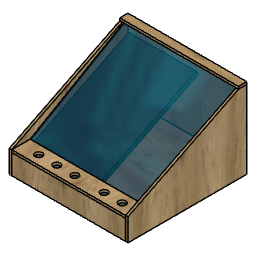
Zeitmaschine (Autodesk Fusion 360 design; units mm, degrees)
Autodesk Fusion 360 part; units mm, degrees
sketch "Skizze1" plane through (0, 0, 0) normal (0, 1, 0) x (1, 0, 0)
  line L0 (0, 0) -> (580, 0)
  line L1 (580, 0) -> (580, 580)
  line L2 (580, 580) -> (0, 580)
  line L3 (0, 580) -> (0, 0)
  line L4 (12, 12) -> (568, 12)
  line L5 (568, 12) -> (568, 568)
  line L6 (568, 568) -> (12, 568)
  line L7 (12, 568) -> (12, 12)
  line L8 (290, 0) -> (290, 580) construction
  dimension "d1" = 580
  dimension "d2" = -12
  constraint horizontal L0
  constraint vertical L1
  constraint horizontal L2
  constraint vertical L3
  constraint coincident L0.start L3.end
  constraint equal L1 L2
  constraint midpoint L0 L8.start
  constraint midpoint L2 L8.end
  measures "d1" distance of L0.end L1.end
sketch "Skizze2" plane through (0, 0, 0) normal (1, 0, 0) x (0, 0, -1)
  line L0 (0, 0) -> (0, 80)
  line L1 (0, 80) -> (100, 80)
  line L2 (100, 80) -> (540, 350)
  line L3 (540, 350) -> (580, 350)
  line L4 (580, 350) -> (580, 0)
  line L5 (580, 0) -> (0, 0)
  line L6 (580, 444.0725) -> (580, 350)
  line L7 (0, 80) -> (540, 350)
  line L8 (0, 80) -> (580, 435.9091)
  line L9 (580, 435.9091) -> (580, 350)
  point P0 (580, 0)
  dimension "d3" = 100
  dimension "d5" = 40
  dimension "d6" = 80
  dimension "d7" = 350
  constraint coincident L0.start L5.end
  constraint vertical L0
  constraint perpendicular L0 L1
  constraint parallel L1 L3
  constraint vertical L4
  constraint coincident P0 L4.end
  constraint perpendicular L3 L6
  constraint parallel L2 L8
  constraint parallel L4 L9
  measures "d3" distance of L0.end L1.end
  measures "d5" distance of L2.end L3.end
  measures "d6" distance of L0.start L0.end
  measures "d7" distance of L3.end P0
extrude "Extrusion1" add sketch "Skizze2" along normal blind 12 contours L0 L1 L2 L3 L4 L5 | L1 L2 L7 makes body 1
ref_plane "Arbeitsebene1" through (290, 0, -290) normal (1, 0, 0) x (0, 0, -1)
mirror "Spiegeln1" about plane through (290, 0, -290) normal (1, 0, 0) of bodies 1 makes body 2
sketch "Skizze3" plane through (0, 0, -580) normal (0, 0, -1) x (-1, 0, 0)
  line L0 (0, 0) -> (0, 350)
  line L1 (0, 350) -> (-12, 350)
  line L2 (-12, 350) -> (-12, 0)
  line L3 (-12, 0) -> (0, 0)
  line L4 (0, 0) -> (-580, 0)
  line L5 (-580, 0) -> (-580, 350)
  line L6 (-580, 350) -> (0, 350)
  line L7 (0, 350) -> (0, 0)
  line L8 (-12, 0) -> (-12, 350)
  line L9 (-568, 0) -> (-568, 350)
  point P0 (-580, 350)
  constraint horizontal L4
  constraint vertical L5
  constraint horizontal L6
  constraint vertical L7
  constraint coincident L0.start L3.end
  constraint coincident P0 L5.end
extrude "Extrusion2" add sketch "Skizze3" against normal blind 12 separate body contours L2 L4 L6 L8 L9 makes body 3
ref_plane "Arbeitsebene2" through (6, 170.2786, -292.3607) normal (0, 0.894427, 0.447214) x (0, -0.447214, 0.894427)
sketch "Skizze7" plane through (6, 170.2786, -292.3607) normal (0, 0.894427, 0.447214) x (0, -0.447214, 0.894427)
  line L0 (241.9063, 17.919) -> (-298.0937, 17.919)
  line L1 (-298.0937, 17.919) -> (-298.0937, 347.919)
  line L2 (-298.0937, 347.919) -> (241.9063, 347.919)
  line L3 (241.9063, 347.919) -> (241.9063, 17.919)
  dimension "d29" = 330
  dimension "d30" = 540
  constraint horizontal L0
  constraint vertical L1
  constraint horizontal L2
  constraint vertical L3
  measures "d29" distance of L0.end L1.end
  measures "d30" distance of L0.start L0.end
extrude "Extrusion7" add sketch "Skizze7" against normal blind 20 separate body makes body 4
sketch "Skizze8" plane through (0, 0, 0) normal (0, -1, 0) x (1, 0, 0)
  line L0 (580, -580) -> (580, 0)
  line L1 (580, 0) -> (568, 0)
  line L2 (568, 0) -> (568, -580)
  line L3 (568, -580) -> (580, -580)
  line L4 (12.3084, -12) -> (568, -12)
  line L5 (568, -12) -> (568, -568)
  line L6 (568, -568) -> (12.3084, -568)
  line L7 (12.3084, -568) -> (12.3084, -12)
  line L8 (12, -568) -> (568, -568)
  dimension "d33" = 12
  constraint horizontal L4
  constraint vertical L5
  constraint horizontal L6
  constraint vertical L7
  constraint coincident L2 L5.end
  constraint coincident L5.end L8
  measures "d33" distance of L1.end L4.end
extrude "Extrusion8" add sketch "Skizze8" against normal blind 12 separate body contours L2 L4 L5 L6 L7 L8 makes body 5
sketch "Skizze9" plane through (0, 0, -12) normal (0, 0, 1) x (1, 0, 0)
  line L0 (12.3084, 0) -> (568, 0)
  line L1 (568, 0) -> (568, 12)
  line L2 (568, 12) -> (12.3084, 12)
  line L3 (12.3084, 12) -> (12.3084, 0)
  line L4 (12.3084, 0) -> (568, 0)
  line L5 (12.3084, 68) -> (12.3084, 0)
  line L6 (568, 68) -> (12.3084, 68)
  line L7 (568, 68) -> (568, 0)
  line L8 (568, 80) -> (568, 0)
  point P0 (568, 80)
  dimension "d41" = 12
  constraint horizontal L4
  constraint vertical L5
  constraint coincident L0 L3.end
  constraint coincident L0.start L3.end
  constraint coincident L5 L6.end
  constraint perpendicular L5 L6
  constraint perpendicular L6 L7
  constraint collinear L7 L8
  measures "d41" distance of P0 L6
extrude "Extrusion9" add sketch "Skizze9" along normal blind 12 separate body makes body 6
sketch "Skizze11" plane through (0, 68, 0) normal (0, 1, 0) x (-1, 0, 0)
  line L0 (-568, -12) -> (-12.3084, -12)
  line L1 (-12.3084, -12) -> (-12.3084, 0)
  line L2 (-12.3084, 0) -> (-568, 0)
  line L3 (-568, 0) -> (-568, -12)
  line L4 (-12.3084, 0) -> (-568, 0)
  line L5 (-568, 0) -> (-568, -90)
  line L6 (-568, -90) -> (-12.3084, -90)
  line L7 (-12.3084, -90) -> (-12.3084, 0)
  line L8 (-568, -540) -> (-568, 0)
  circle A0 centre (-99.0921, -45) radius 17.4859
  circle A1 centre (-187.2764, -45) radius 17.4859
  circle A2 centre (-275.4607, -45) radius 17.4859
  circle A3 centre (-418.767, -45) radius 17.4859
  circle A4 centre (-506.9513, -45) radius 17.4859
  line L9 (-99.0921, -90) -> (-99.0921, 0) construction
  line L10 (-99.0921, -45) -> (-187.2764, -45) construction
  line L11 (-187.2764, -45) -> (-275.4607, -45) construction
  line L12 (-418.767, -45) -> (-506.9513, -45) construction
  line L13 (-290.1542, -90) -> (-290.1542, -320)
  dimension "d42" = 90
  constraint horizontal L4
  constraint vertical L5
  constraint horizontal L6
  constraint vertical L7
  constraint coincident L1.end L2.start
  constraint collinear L5 L8
  constraint equal A3 A4
  constraint equal A2 A3
  constraint equal A1 A2
  constraint equal A0 A1
  constraint coincident L6 L9.start
  constraint coincident L4 L9.end
  constraint perpendicular L4 L9
  constraint coincident A0.centre L9
  constraint midpoint A0.centre L9
  constraint coincident A0.centre L10.start
  constraint coincident A1.centre L10.end
  constraint coincident A2.centre L11.end
  constraint horizontal L11
  constraint coincident A3.centre L12.start
  constraint coincident A4.centre L12.end
  constraint horizontal L10
  constraint equal L10 L11
  constraint equal L11 L12
  constraint collinear L11 L12
  constraint midpoint L6 L13.start
  constraint perpendicular L6 L13
  measures "d42" distance of L2.end L5.end
extrude "Extrusion11" add sketch "Skizze11" along normal blind 12 separate body makes body 7
sketch "Skizze12" plane through (568, 0, 0) normal (-1, 0, 0) x (0, 0, 1)
  line L0 (0, 0) -> (0, 80)
  line L1 (0, 80) -> (-540, 350)
  line L2 (-540, 350) -> (-580, 350)
  line L3 (-580, 350) -> (-580, 0)
  line L4 (-580, 0) -> (0, 0)
  line L5 (-90, 80) -> (-614.609, 383.9864)
  line L6 (-93.0082, 74.8086) -> (-617.6172, 378.795)
  line L7 (-90, 80) -> (-93.0082, 74.8086)
  line L8 (-614.609, 383.9864) -> (-617.6172, 378.795)
  line L9 (-90, 80) -> (-5.2713, 30.9037)
  line L10 (-93.0082, 74.8086) -> (-8.2795, 25.7123)
  line L11 (-5.2713, 30.9037) -> (-8.2795, 25.7123)
  point P0 (-90, 80)
  dimension "d45" = 6
  dimension "d46" = 8
  constraint parallel L5 L6
  constraint perpendicular L5 L7
  constraint perpendicular L5 L8
  constraint coincident P0 L5.start
  constraint perpendicular L7 L9
  constraint perpendicular L7 L10
  constraint perpendicular L10 L11
  measures "d45" distance of P0 L6.start
  measures "d46" distance of L1.end L5
extrude "Extrusion12" cut sketch "Skizze12" against normal blind 5 contours L2 L5 L6 L7 | L7 L9 L10 L11 bodies 2
sketch "Skizze13" plane through (0, 350, 0) normal (0, 1, 0) x (-1, 0, 0)
  line L0 (-573, -555.9565) -> (-568, -555.9565)
  line L1 (-568, -555.9565) -> (-568, -540)
  line L2 (-568, -540) -> (-580, -540)
  line L3 (-580, -540) -> (-580, -580)
  line L4 (-580, -580) -> (-568, -580)
  line L5 (-568, -580) -> (-568, -567.9238)
  line L6 (-568, -567.9238) -> (-573, -567.9238)
  line L7 (-573, -567.9238) -> (-573, -555.9565)
  line L8 (0, -580) -> (-580, -580)
  line L9 (-580, -580) -> (-580, -540)
  line L10 (-580, -540) -> (0, -540)
  line L11 (0, -540) -> (0, -580)
  constraint horizontal L8
  constraint vertical L9
  constraint horizontal L10
  constraint vertical L11
  constraint coincident L2.end L3.start
extrude "Extrusion13" add sketch "Skizze13" along normal blind 12 separate body makes body 8
extrude "Extrusion14" add 1 faces at (573, 241.9041, -377.3866) along direction (-1, 0, 0) blind 561 separate body on bodies 2 makes body 9
sketch "Skizze14" plane through (0, 12, 0) normal (0, 1, 0) x (-1, 0, 0)
  line L0 (-568, -568) -> (-12.3084, -568)
  line L1 (-12.3084, -568) -> (-12.3084, -12)
  line L2 (-12.3084, -12) -> (-568, -12)
  line L3 (-568, -12) -> (-568, -568)
  circle A0 centre (-460, -420) radius 78.7452
extrude "Extrusion15" add sketch "Skizze14" along normal blind 100 separate body contours A0 makes body 10
extrude "Extrusion16" add 2 faces at (197.539, 0, -4) (197.3333, 0, -576) along direction (0, -1, 0) blind 30 separate body on bodies 3 6 makes body 11 at (197.539, -10, -12) makes body 12 at (197.3333, -10, -580)
extrude "Extrusion17" add 2 faces at (576, 0, -386.6667) (4, 0, -386.6667) along direction (0, -1, 0) blind 30 separate body on bodies 1 2 makes body 13 at (580, -20, -386.6667) makes body 14 at (0, -20, -386.6667)
combine "Kombinieren1" operation add target body 1 tool bodies 14
combine "Kombinieren2" operation add target body 6 tool bodies 11
combine "Kombinieren3" operation add target body 2 tool bodies 13
combine "Kombinieren4" operation add target body 3 tool bodies 12
sketch "Skizze15" plane through (0, 0, 0) normal (0, 0, 1) x (1, 0, 0)
hidden bodies 10
named bodies: "linke Wand", "rechte Wand", "hintere Wand", "TV", "Boden", "Front", "Ablage Knoepfe", "oben Abdeckung", "glass", "podest"
